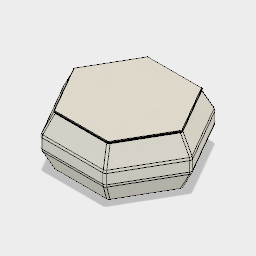
Momoyama v2 (Autodesk Fusion 360 design; units mm, degrees)
Autodesk Fusion 360 part; units mm, degrees
sketch "Sketch1" plane through (0, 0, 0) normal (0, 1, 0) x (1, 0, 0)
  line L0 (48.4974, -84) -> (96.9948, 0)
  line L1 (96.9948, 0) -> (48.4974, 84)
  line L2 (48.4974, 84) -> (-48.4974, 84)
  line L3 (-48.4974, 84) -> (-96.9948, 0)
  line L4 (-96.9948, 0) -> (-48.4974, -84)
  line L5 (-48.4974, -84) -> (48.4974, -84)
  dimension "d1" = 84
  measures "d1" distance of origin L5
extrude "Extrude1" add sketch "Sketch1" along normal blind 32 draft 25 makes body 1
ref_plane "WorkPlane1" through (0, 32, 0) normal (0, 1, 0) x (1, 0, 0)
mirror "Mirror1" about plane through (0, 32, 0) normal (0, 1, 0) of bodies 1 makes body 2
move_body "Move1" bodies 2 to x (1, 0, 0) y (0, 1, 0) z (0, 0, 1) at (0, 320, 0)
extrude "Extrude2" add 1 faces at (19.0375, 32, 32.9739) along direction (0, 1, 0) blind 22 on bodies 1 bodies 1
move_body "Move2" bodies 2 to x (1, 0, 0) y (0, 1, 0) z (0, 0, 1) at (0, -298, 0)
combine "Combine1" operation add target body 1 tool bodies 2
sketch "Sketch2" plane through (0, 86, 0) normal (0, 1, 0) x (-1, 0, 0)
  line L0 (48.4974, 84) -> (-48.4974, 84)
  line L1 (-48.4974, 84) -> (-96.9948, 0)
  line L2 (-96.9948, 0) -> (-48.4974, -84)
  line L3 (-48.4974, -84) -> (48.4974, -84)
  line L4 (48.4974, -84) -> (96.9948, 0)
  line L5 (96.9948, 0) -> (48.4974, 84)
  line L6 (-46.188, 80) -> (-92.376, 0)
  line L7 (-92.376, 0) -> (-46.188, -80)
  line L8 (-46.188, -80) -> (46.188, -80)
  line L9 (46.188, -80) -> (92.376, 0)
  line L10 (92.376, 0) -> (46.188, 80)
  line L11 (46.188, 80) -> (-46.188, 80)
  line L12 (-48.4974, 84) -> (-96.9948, 0)
  line L13 (-96.9948, 0) -> (-48.4974, -84)
  line L14 (-48.4974, -84) -> (48.4974, -84)
  line L15 (48.4974, -84) -> (96.9948, 0)
  line L16 (96.9948, 0) -> (48.4974, 84)
  line L17 (48.4974, 84) -> (-48.4974, 84)
extrude "Extrude3" cut sketch "Sketch2" against normal blind 80 contours L6 L7 L8 L9 L10 L11 bodies 1
ref_plane "WorkPlane2" through (0, 83, 0) normal (0, 1, 0) x (-1, 0, 0)
sketch "Sketch3" plane through (0, 83, 0) normal (0, 1, 0) x (1, 0, 0)
  line L0 (-46.188, 80) -> (-92.376, 0)
  line L1 (-92.376, 0) -> (-46.188, -80)
  line L2 (-46.188, -80) -> (46.188, -80)
  line L3 (46.188, -80) -> (92.376, 0)
  line L4 (92.376, 0) -> (46.188, 80)
  line L5 (46.188, 80) -> (-46.188, 80)
extrude "Extrude4" add sketch "Sketch3" along normal blind 3 separate body makes body 3
ref_plane "WorkPlane3" through (0, 86, 0) normal (0, 1, 0) x (0, 0, 1)
sketch "Sketch4" plane through (0, 86, 0) normal (0, 1, 0) x (1, 0, 0)
  line L0 (48.4974, -84) -> (96.9948, 0)
  line L1 (96.9948, 0) -> (48.4974, 84)
  line L2 (48.4974, 84) -> (-48.4974, 84)
  line L3 (-48.4974, 84) -> (-96.9948, 0)
  line L4 (-96.9948, 0) -> (-48.4974, -84)
  line L5 (-48.4974, -84) -> (48.4974, -84)
extrude "Extrude5" add sketch "Sketch4" along normal blind 3 bodies 3
fillet "Fillet1" radius 10 6 edges at (-85.6688, 54, -49.4609) (0, 54, -98.9218) (-85.6688, 54, 49.4609) (0, 54, 98.9218) (85.6688, 54, 49.4609) (85.6688, 54, -49.4609) on bodies 1
fillet "Fillet2" radius 10 6 edges at (85.6688, 32, -49.4609) (85.6688, 32, 49.4609) (0, 32, -98.9218) (-85.6688, 32, -49.4609) (-85.6688, 32, 49.4609) (0, 32, 98.9218) on bodies 1
fillet "Fillet3" radius 5 30 edges at (52.5345, 71.0046, 90.9925) (56.9757, 53.9474, 98.6848) (57.1126, 43, 98.9218) (56.9757, 32.0526, 98.6848) (52.5345, 14.9954, 90.9925) (-52.5345, 71.0046, 90.9925) (-56.9757, 53.9474, 98.6848) (-57.1126, 43, 98.9218) (-56.9757, 32.0526, 98.6848) (-52.5345, 14.9954, 90.9925) (-105.069, 71.0046, 0) (-113.9514, 53.9474, 0) (-114.2251, 43, 0) (-113.9514, 32.0526, 0) (-105.069, 14.9954, 0) (105.069, 71.0046, 0) (113.9514, 53.9474, 0) (114.2251, 43, 0) (113.9514, 32.0526, 0) (105.069, 14.9954, 0) (52.5345, 71.0046, -90.9925) (56.9757, 53.9474, -98.6848) (57.1126, 43, -98.9218) (56.9757, 32.0526, -98.6848) (52.5345, 14.9954, -90.9925) (-52.5345, 71.0046, -90.9925) (-56.9757, 53.9474, -98.6848) (-57.1126, 43, -98.9218) (-56.9757, 32.0526, -98.6848) (-52.5345, 14.9954, -90.9925) on bodies 1
fillet "Fillet4" radius 1 12 edges at (72.7461, 89, 42) (72.7461, 86, 42) (72.7461, 86, -42) (72.7461, 89, -42) (0, 89, -84) (0, 86, -84) (-72.7461, 86, -42) (-72.7461, 89, -42) (-72.7461, 86, 42) (-72.7461, 89, 42) (0, 89, 84) (0, 86, 84) on bodies 3
named bodies: "body", "lead"
